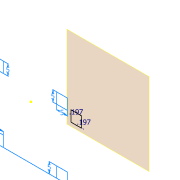
# Autodesk Inventor part: ServoHolderColumns
Saved by Autodesk Inventor 2018 (Build 220112000, 112)
## iProperties
Created: 2018-10-17
Part Number: ServoHolderColumns
Material: Generic
Document SubType Name: Modeling
Designer: Vulnic
Density: 1 g/cm^3
Appearance: Default
Author: Vulnic
Autodesk Inventor part; units mm, degrees
ref_plane "YZ Plane" through (0, 0, 0) normal (1, 0, 0) x (0, 1, 0)
ref_plane "XZ Plane" through (0, 0, 0) normal (0, 1, 0) x (-1, 0, 0)
ref_plane "XY Plane" through (0, 0, 0) normal (0, 0, 1) x (1, 0, 0)
ref_plane "Work Plane1" through (36.1477, 18.6279, -6.7668) normal (0, 0, 1) x (1, 0, 0)
sketch "Sketch1" plane through (36.1477, 18.6279, -6.7668) normal (0, 0, 1) x (1, 0, 0)
  line L0 (-17.5, -17.5) -> (17.5, -17.5) projected
  line L1 (17.5, -17.5) -> (17.5, 17.5) projected
  line L2 (17.5, 17.5) -> (-17.5, 17.5) projected
  line L3 (-17.5, 17.5) -> (-17.5, -17.5) projected
  line L4 (-17.5, -17.5) -> (17.5, -17.5) projected
  line L5 (17.5, -17.5) -> (17.5, 17.5) projected
  line L6 (17.5, 17.5) -> (-17.5, 17.5) projected
  line L7 (-17.5, 17.5) -> (-17.5, -17.5) projected
  line L8 (-17.5, -17.5) -> (17.5, -17.5) projected
  line L9 (17.5, -17.5) -> (17.5, 17.5) projected
  line L10 (17.5, 17.5) -> (-17.5, 17.5) projected
  line L11 (-17.5, 17.5) -> (-17.5, -17.5) projected
  line L12 (17.5, -17.5) -> (12.5, -17.5)
  line L13 (12.5, -17.5) -> (12.5, -12.5)
  line L14 (12.5, -12.5) -> (17.5, -12.5)
  line L15 (17.5, -12.5) -> (17.5, -17.5)
  line L16 (-17.5, -17.5) -> (-12.5, -17.5)
  line L17 (-12.5, -17.5) -> (-12.5, -12.5)
  line L18 (-12.5, -12.5) -> (-17.5, -12.5)
  line L19 (-17.5, -12.5) -> (-17.5, -17.5)
  line L20 (-17.5, 17.5) -> (-12.5, 17.5)
  line L21 (-12.5, 17.5) -> (-12.5, 12.5)
  line L22 (-12.5, 12.5) -> (-17.5, 12.5)
  line L23 (-17.5, 12.5) -> (-17.5, 17.5)
  line L24 (17.5, 17.5) -> (12.5, 17.5)
  line L25 (12.5, 17.5) -> (12.5, 12.5)
  line L26 (12.5, 12.5) -> (17.5, 12.5)
  line L27 (17.5, 12.5) -> (17.5, 17.5)
  point P0 (-36.1477, -18.6279)
  dimension "d2" = 5
  dimension "d3" = 5
  dimension "d4" = 5
  dimension "d5" = 5
  constraints: 32 end point, 12 parallel, 4 horizontal, 4 perpendicular
  measures "d2" distance of L13.end L14.end
  measures "d3" distance of L16.end L17.end
  measures "d4" distance from line of L3 L17.end
  measures "d5" distance of L21.end L20.end
extrude "Extrusion1" add sketch "Sketch1" along normal blind 60 contours L3 L18 L17 L0 | L13 L14 L1 L0 | L3 L2 L21 L22 | L26 L25 L2 L1
body "Solid1"
